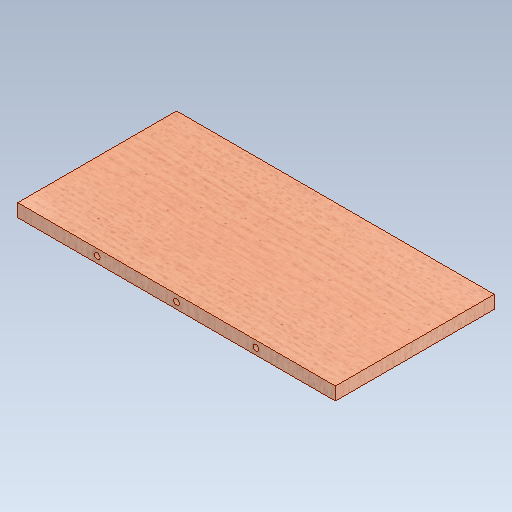
# Autodesk Inventor part: BasePC
Saved by Autodesk Inventor 2020.3 (Build 243373000, 373)
## iProperties
Created: 2020-10-29
Part Number: BasePC
Material: Madera (roble)
Document SubType Name: Modeling
Designer: codig
Density: 0.76 g/cm^3
Appearance: Roble blanco - Natural brillo medio
Mass: 1316.2 g
Surface Area: 2226.38 cm^2
Volume: 1731.84 cm^3
Author: codig
Autodesk Inventor part; units mm, degrees
ref_plane "YZ Plane" through (0, 0, 0) normal (1, 0, 0) x (0, 1, 0)
ref_plane "XZ Plane" through (0, 0, 0) normal (0, 1, 0) x (-1, 0, 0)
ref_plane "XY Plane" through (0, 0, 0) normal (0, 0, 1) x (1, 0, 0)
sketch "Boceto1" plane through (0, 0, 0) normal (0, 1, 0) x (-1, 0, 0)
  line L0 (100, -100) -> (540, -100)
  line L1 (540, -100) -> (540, -320)
  line L2 (540, -320) -> (100, -320)
  line L3 (100, -320) -> (100, -100)
  point P0 (0, 0)
  constraints: 8 end point, 2 parallel, 1 horizontal, 1 perpendicular
extrude "Extrusión1" add sketch "Boceto1" along normal blind 18
sketch "Boceto2" plane through (-540, 0, -100) normal (0, 0, 1) x (1, 0, 0)
  line L0 (0, 0) -> (0, 18) projected
  circle A0 centre (330, 9) radius 4
  circle A1 centre (220, 9) radius 4
  circle A2 centre (110, 9) radius 4
  point P0 (540, 0)
  constraints: 3 centre point
hole "Agujero1" at (-430, 9, -100) at (-320, 9, -100) at (-210, 9, -100) direction (0, 0, -1) diameter 8 depth 35
sketch "Boceto3" plane through (-100, 0, -320) normal (0, 0, -1) x (-1, 0, 0)
  line L0 (0, 0) -> (0, 18) projected
  circle A0 centre (110, 9) radius 4 projected
  circle A1 centre (110, 9) radius 4
  circle A2 centre (220, 9) radius 4
  circle A3 centre (330, 9) radius 4
  point P0 (-100, 0)
  constraints: 3 centre point, 1 coincident
hole "Agujero2" at (-210, 9, -320) at (-320, 9, -320) at (-430, 9, -320) direction (0, 0, 1) diameter 8 depth 35
